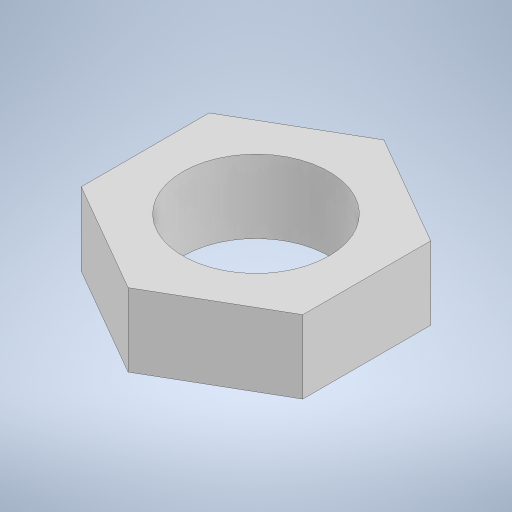
# Autodesk Inventor part: M2Nut
Saved by Autodesk Inventor 2024.2 (Build 282272000, 272)
## iProperties
Created: 2024-05-04
Part Number: M2Nut
Material: Generic
Document SubType Name: Modeling
Designer: ringl
Density: 1 g/cm^3
Appearance: Default
Author: ringl
Autodesk Inventor part; units mm, degrees
ref_plane "YZ Plane" through (0, 0, 0) normal (1, 0, 0) x (0, 1, 0)
ref_plane "XZ Plane" through (0, 0, 0) normal (0, 1, 0) x (-1, 0, 0)
ref_plane "XY Plane" through (0, 0, 0) normal (0, 0, 1) x (1, 0, 0)
sketch "Sketch1" plane through (0, 0, 0) normal (0, 1, 0) x (-1, 0, 0)
  line L0 (0, -1.75) -> (-1.5155, -0.875)
  line L1 (-1.5155, -0.875) -> (-1.5155, 0.875)
  line L2 (-1.5155, 0.875) -> (0, 1.75)
  line L3 (0, 1.75) -> (1.5155, 0.875)
  line L4 (1.5155, 0.875) -> (1.5155, -0.875)
  line L5 (1.5155, -0.875) -> (0, -1.75)
  circle A0 centre (0, 0) radius 1
  dimension "d0" = 2
  dimension "d1" = 3.5
  constraints: 12 end point, 2 coincident, 1 centre point, 1 vertical alignment, 13 other
  measures "d0" diameter of A0
  measures "d1" distance of L0.start L2.end
extrude "Extrusion1" add sketch "Sketch1" along normal blind 1
body "Solid1"
